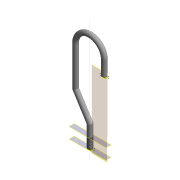
# Autodesk Inventor part: hook prototype
Saved by Autodesk Inventor 2013 (Build 170138000, 138)
## iProperties
Created: 2013-12-21
Part Number: hook prototype
Material: Generic
Document SubType Name: Modeling
Designer: kahohbein
Density: 1 g/cm^3
Author: kahohbein
Autodesk Inventor part; units mm, degrees
ref_plane "YZ Plane" through (0, 0, 0) normal (1, 0, 0) x (0, 1, 0)
ref_plane "XZ Plane" through (0, 0, 0) normal (0, 1, 0) x (-1, 0, 0)
sketch "Sketch1" plane through (0, 0, 0) normal (0, 0, 1) x (1, 0, 0)
  line L0 (19.05, 0) -> (19.05, 25.4)
  line L1 (19.05, 25.4) -> (0, 55.8663)
  arc A0 (38.1, 107.95) -> (0, 107.95) centre (19.05, 107.95) ccw
  line L2 (0, 55.8663) -> (0, 107.95)
  line L3 (38.1, 88.9) -> (38.1, 107.95)
  point P0 (0, 0)
  dimension "d2" = 25.4
  constraints: 8 end point, 2 point on circle, 1 centre point, 1 parallel, 1 tangent
  measures "d2" distance of L0.start L0.end
ref_plane "Work Plane1" through (19.05, 0, 0) normal (0, 1, 0) x (-1, 0, 0)
sketch "Sketch2" plane through (19.05, 0, 0) normal (0, 1, 0) x (-1, 0, 0)
  circle A0 centre (0, 0) radius 3.175
  point P0 (19.05, 0)
  dimension "d6" = 6.35
  constraints: 1 centre point
  measures "d6" diameter of A0
sweep "Sweep1" add profiles "Sketch2" path "Sketch1"
sketch "Sketch3" plane through (19.05, 0, 0) normal (0, 1, 0) x (-1, 0, 0)
  circle A0 centre (0, 0) radius 3.175
  point P0 (19.05, 0)
  dimension "d8" = 6.35
  constraints: 1 centre point
  measures "d8" diameter of A0
extrude "Extrusion1" add sketch "Sketch3" against normal blind 3.175
ref_plane "Work Plane3" through (19.05, 11.1125, 0) normal (0, -1, 0) x (1, 0, 0)
ref_plane "Work Plane2" through (19.05, -3.175, 0) normal (0, -1, 0) x (1, 0, 0)
split_face "Split1"
thread "Thread1" size "1/4-20 UNC" class "2A" standard "ANSI Unified Screw Threads" full length
sketch "Sketch4" plane through (38.1, 88.9, 0) normal (0, -1, 0) x (1, 0, 0)
  circle A0 centre (0, 0) radius 3.175 projected
  point P0 (-38.1, 0)
  point P1 (3.175, 0)
  point P2 (-3.1732, -0.1068)
  constraints: 2 point on circle
sketch "Sketch5" plane through (19.05, -3.175, 0) normal (0, -1, 0) x (1, 0, 0)
  circle A0 centre (0, 0) radius 3.175 projected
  point P0 (-19.05, 0)
  point P1 (3.175, 0)
  constraints: 1 horizontal alignment, 1 other
ref_plane "Work Plane6" through (41.275, 88.9, 0) normal (-0.0168, 0.0035, 0.9999) x (-0.9999, 0, -0.0168)
body "Solid1"
